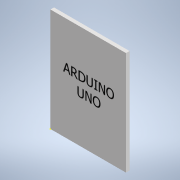
# Autodesk Inventor part: arduino_sketch
Saved by Autodesk Inventor 2020 (Build 240168000, 168)
## iProperties
Created: 2019-10-22
Part Number: arduino_sketch
Material: Generic
Document SubType Name: Modeling
Designer: Connor
Density: 1 g/cm^3
Appearance: Default
Author: Connor
Autodesk Inventor part; units mm, degrees
ref_plane "YZ Plane" through (0, 0, 0) normal (1, 0, 0) x (0, 1, 0)
ref_plane "XZ Plane" through (0, 0, 0) normal (0, 1, 0) x (-1, 0, 0)
ref_plane "XY Plane" through (0, 0, 0) normal (0, 0, 1) x (1, 0, 0)
sketch "Sketch1" plane through (0, 0, 0) normal (0, 0, 1) x (1, 0, 0)
  line L0 (0, 0) -> (0, 73.025)
  line L1 (0, 73.025) -> (53.34, 73.025)
  line L2 (53.34, 73.025) -> (53.34, 0)
  line L3 (53.34, 0) -> (0, 0)
  dimension "d0" = 73.025
  dimension "d1" = 53.34
  constraints: 8 end point, 3 perpendicular, 1 vertical
  measures "d0" distance of L0.start L0.end
  measures "d1" distance of L0.end L1.end
extrude "Extrusion1" add sketch "Sketch1" along normal blind 2.54
sketch "Sketch2" plane through (0, 0, 2.54) normal (0, 0, 1) x (1, 0, 0)
  line L0 (9.1778, 46.027) -> (44.9714, 46.027) construction
  line L1 (44.9714, 46.027) -> (44.9714, 12.4361) construction
  line L2 (44.9714, 12.4361) -> (9.1778, 12.4361) construction
  line L3 (9.1778, 12.4361) -> (9.1778, 46.027) construction
  point P0 (0, 0)
  constraints: 2 other
body "Solid1"
